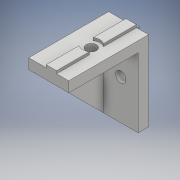
# Autodesk Inventor part: Estrutura - SuporteCanto
Saved by Autodesk Inventor 2017 (Build 210142000, 142)
## iProperties
Created: 2020-10-04
Part Number: Estrutura - SuporteCanto
Material: Generic
Document SubType Name: Modeling
Designer: ale
Density: 1 g/cm^3
Appearance: Default
Author: ale
Autodesk Inventor part; units mm, degrees
ref_plane "YZ Plane" through (0, 0, 0) normal (1, 0, 0) x (0, 1, 0)
ref_plane "XZ Plane" through (0, 0, 0) normal (0, 1, 0) x (-1, 0, 0)
ref_plane "XY Plane" through (0, 0, 0) normal (0, 0, 1) x (1, 0, 0)
sketch "Sketch1" plane through (0, 0, 0) normal (0, 0, 1) x (1, 0, 0)
  line L0 (0, 6) -> (0, -40)
  line L1 (-20, 6) -> (-20, -40)
  line L2 (-20, 6) -> (0, 6)
  line L3 (-20, -40) -> (0, -40)
  point P0 (0, 0)
  dimension "d6" = 20
  dimension "d10" = 6
  constraints: 8 end point, 2 horizontal, 1 parallel, 1 point on line, 1 vertical
  measures "d6" distance between parallel lines of L0 L1
  measures "d10" distance from line of point (0, 0) L2
extrude "Extrusion1" add sketch "Sketch1" against normal blind 6
sketch "Sketch2" plane through (0, 0, -6) normal (0, 0, -1) x (-1, 0, 0)
  line L0 (20, -40) -> (20, 6) projected
  line L1 (0, 6) -> (0, -40) projected
  line L2 (20, 6) -> (0, 6)
  line L3 (0, 6) -> (0, 0)
  line L4 (0, 0) -> (20, 0)
  line L5 (20, 0) -> (20, 6)
  point P0 (0, 0)
  dimension "d13" = 6
  constraints: 8 end point, 2 parallel, 1 horizontal, 1 perpendicular, 1 point on line
  measures "d13" distance of L3.end L2.end
extrude "Extrusion2" add sketch "Sketch2" along normal blind 40
sketch "Sketch3" plane through (0, 0, 0) normal (0, 0, 1) x (1, 0, 0)
  line L0 (0, 6) -> (-20, 6) projected
  line L1 (-13, 6) -> (-13, -40)
  line L2 (-20, 6) -> (-20, -40) projected
  line L3 (-7, 6) -> (-7, -40)
  line L4 (0, -40) -> (-20, -40) projected
  line L5 (-13, 6) -> (-7, 6)
  line L6 (-13, -40) -> (-7, -40)
  point P0 (0, 0)
  dimension "d16" = 7
  dimension "d17" = 6
  constraints: 8 end point, 3 point on line, 2 collinear, 1 perpendicular, 1 vertical
  measures "d16" distance between parallel lines of L1 L2
  measures "d17" distance between parallel lines of L3 L1
extrude "Extrusion3" add sketch "Sketch3" along normal blind 1.5 contours L3 L4 L1 L0
sketch "Sketch4" plane through (-20, 6, -46) normal (0, 1, 0) x (1, 0, 0)
  line L0 (20, -46) -> (13, -46) projected
  line L1 (13, -46) -> (13, 0)
  line L2 (20, 0) -> (0, 0) projected
  line L3 (7, -46) -> (7, -47.5) projected
  line L4 (7, -46) -> (7, 0)
  line L5 (7, 0) -> (13, 0)
  line L6 (7, -46) -> (13, -46)
  constraints: 8 end point, 2 perpendicular, 2 vertical, 1 point on line
extrude "Extrusion4" add sketch "Sketch4" along normal blind 1.5
sketch "Sketch5" plane through (-20, 7.5, -46) normal (0, 1, 0) x (1, 0, 0)
  line L0 (20, -46) -> (20, 0) projected
  line L1 (0, 0) -> (7, 0) projected
  point P0 (10, -23)
  dimension "d22" = 10
  dimension "d23" = 23
  measures "d22" distance from line of L0 point (10, -23)
  measures "d23" distance from line of L1 point (10, -23)
hole "Hole1" at (-10, 7.5, -23) direction (0, -1, 0) diameter 6 end through all counterbore diameter 10 counterbore depth 1.5
sketch "Sketch6" plane through (0, 0, 1.5) normal (0, 0, 1) x (1, 0, 0)
  line L0 (-7, -40) -> (0, -40) projected
  line L1 (0, -40) -> (0, 6) projected
  point P0 (0, 0)
  point P1 (-10, -17)
  dimension "d31" = 23
  dimension "d32" = 10
  measures "d31" distance from line of L0 point (-10, -17)
  measures "d32" distance from line of L1 point (-10, -17)
hole "Hole2" at (-10, -17, 1.5) direction (0, 0, -1) diameter 6 end through all counterbore diameter 10 counterbore depth 1.5
sketch "Sketch7" plane through (-20, -40, 0) normal (-1, 0, 0) x (0, 0, 1)
  line L0 (0, 0) -> (0, 46) projected
  line L1 (0, 46) -> (-46, 46) projected
  line L2 (0, 0) -> (0, 46)
  line L3 (-46, 46) -> (-46, 40) projected
  line L4 (0, 46) -> (-46, 46)
  line L5 (-46, 46) -> (-46, 40)
  line L6 (0, 0) -> (-6, 0) projected
  line L7 (-46, 40) -> (-6, 0)
  line L8 (-6, 0) -> (0, 0)
  point P0 (0, 40)
  constraints: 10 end point, 2 perpendicular, 1 collinear, 1 vertical
extrude "Extrusion5" add sketch "Sketch7" along normal blind 3
body "Solid1"
